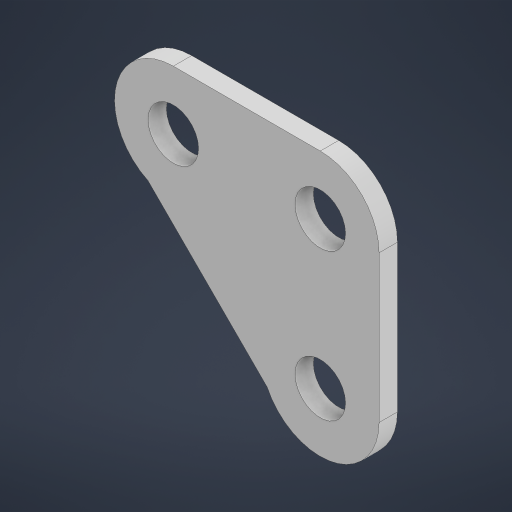
# Autodesk Inventor part: Wing poly connection 2
Saved by Autodesk Inventor 2023.4 (Build 274418000, 418)
## iProperties
Created: 2024-01-15
Part Number: Wing poly connection 2
Material: Generic
Document SubType Name: Modeling
Designer: diego
Density: 1 g/cm^3
Appearance: Default
Author: diego
Autodesk Inventor part; units mm, degrees
ref_plane "YZ Plane" through (0, 0, 0) normal (1, 0, 0) x (0, 1, 0)
ref_plane "XZ Plane" through (0, 0, 0) normal (0, 1, 0) x (-1, 0, 0)
ref_plane "XY Plane" through (0, 0, 0) normal (0, 0, 1) x (1, 0, 0)
sketch "Sketch1" plane through (0, 0, 0) normal (0, 0, 1) x (1, 0, 0)
  circle A0 centre (0, 0) radius 2.1844
  line L0 (0, 0) -> (12.7, 0)
  circle A1 centre (12.7, 0) radius 2.1844
  line L1 (12.7, 0) -> (12.7, -12.7)
  circle A2 centre (12.7, -12.7) radius 2.1844
  circle A3 centre (0, 0) radius 5.08
  circle A4 centre (12.7, 0) radius 5.08
  circle A5 centre (12.7, -12.7) radius 5.08
  line L2 (0, 5.08) -> (12.7, 5.08)
  line L3 (17.78, 0) -> (17.78, -12.7)
  line L4 (-4.5864, -2.1844) -> (8.1136, -14.8844)
  point P0 (-2.1844, -4.5864)
  dimension "d8" = 4.3688
  dimension "d9" = 12.7
  dimension "d10" = 4.3688
  dimension "d11" = 12.7
  dimension "d12" = 4.3688
  dimension "d13" = 10.16
  dimension "d14" = 10.16
  dimension "d15" = 10.16
  constraints: 10 end point, 6 centre point, 6 point on circle, 5 coincident, 2 tangent, 1 horizontal, 1 vertical
  measures "d8" diameter of A0
  measures "d9" distance of L0.start L0.end
  measures "d10" diameter of A1
  measures "d11" distance of L1.start L1.end
  measures "d12" diameter of A2
  measures "d13" diameter of A3
  measures "d14" diameter of A4
  measures "d15" diameter of A5
extrude "Extrusion2" add sketch "Sketch1" along normal blind 1.5875 contours A3 L2 A4 L0 | A3 L4 | L0 A4 L1 A5 L4 A3 | A4 L1 A1 L0 | L0 A1 L1 A4 | A3 L4 | A4 L3 A5 L1 | A5
body "Solid2"
